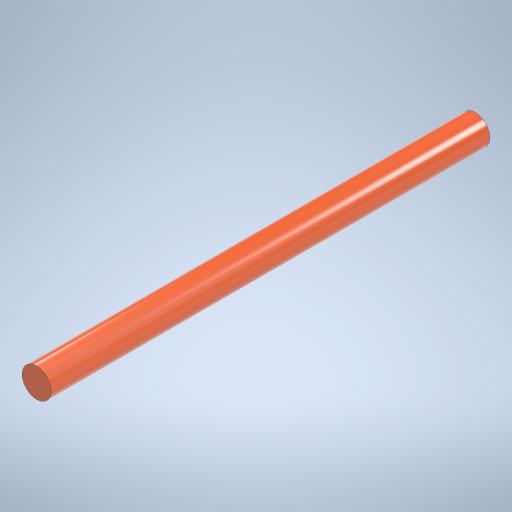
# Autodesk Inventor part: rodante
Saved by Autodesk Inventor 2023 (Build 270158030, 158C)
## iProperties
Created: 2022-05-25
Part Number: rodante
Material: Genérico
Document SubType Name: Modeling
Designer: isaac
Density: 1 g/cm^3
Appearance: Valor por defecto
Author: isaac
Autodesk Inventor part; units mm, degrees
ref_plane "YZ Plane" through (0, 0, 0) normal (1, 0, 0) x (0, 1, 0)
ref_plane "XZ Plane" through (0, 0, 0) normal (0, 1, 0) x (-1, 0, 0)
ref_plane "XY Plane" through (0, 0, 0) normal (0, 0, 1) x (1, 0, 0)
sketch "Boceto2" plane through (0, 0, 0) normal (0, 0, 1) x (1, 0, 0)
  circle A0 centre (0, 0) radius 50
  dimension "d0" = 100
  constraints: 1 centre point, 1 coincident
  measures "d0" diameter of A0
extrude "Extrusión1" add sketch "Boceto2" along normal mid plane 1500
